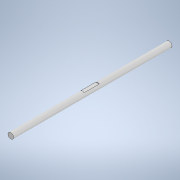
# Autodesk Inventor part: Eje_Engranes_llanta
Saved by Autodesk Inventor 2021 (Build 250183000, 183)
## iProperties
Created: 2021-02-06
Part Number: Eje_Engranes_llanta
Material: Genérico
Document SubType Name: Modeling
Designer: rotje
Density: 1 g/cm^3
Appearance: Valor por defecto
Author: rotje
Autodesk Inventor part; units mm, degrees
ref_plane "YZ Plane" through (0, 0, 0) normal (1, 0, 0) x (0, 1, 0)
ref_plane "XZ Plane" through (0, 0, 0) normal (0, 1, 0) x (-1, 0, 0)
ref_plane "XY Plane" through (0, 0, 0) normal (0, 0, 1) x (1, 0, 0)
sketch "Boceto1" plane through (0, 0, 0) normal (0, 0, 1) x (1, 0, 0)
  circle A0 centre (0, 0) radius 7.5
  dimension "d0" = 15
  constraints: 1 centre point, 1 coincident
  measures "d0" diameter of A0
extrude "Extrusión1" add sketch "Boceto1" along normal mid plane 420
sketch "Boceto3" plane through (0, 0, 0) normal (0, 0, 1) x (1, 0, 0)
  circle A0 centre (0, 0) radius 7.5 projected
  line L0 (0, 0) -> (0, 7.5)
  line L1 (0, 7.5) -> (0, 6)
  line L2 (0, 6) -> (4.5, 6)
  line L3 (4.5, 6) -> (-4.5, 6)
  arc A1 (4.5, 6) -> (-4.5, 6) centre (0, 0) ccw
  dimension "d6" = 1.5
  constraints: 8 end point, 6 point on circle, 2 point on line, 1 centre point, 1 perpendicular, 1 vertical
  measures "d6" distance of L0.end L1.end
extrude "Extrusión3" cut sketch "Boceto3" along normal mid plane 40 contours L2 L0 A0 | A0 L0 L3
